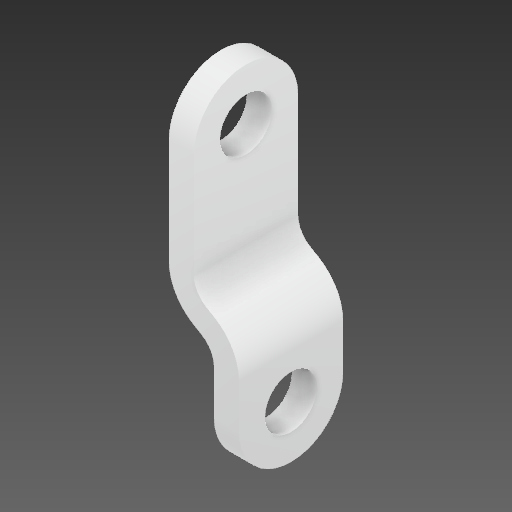
# Autodesk Inventor part: ForearmActuatorConnector2
Saved by Autodesk Inventor 2020 (Build 240168000, 168)
## iProperties
Created: 2020-04-15
Part Number: ForearmActuatorConnector2
Material: Aluminum 6061
Document SubType Name: Sheet Metal
Designer: valer
Density: 2.7 g/cm^3
Sheet Metal Rule: Default
Appearance: Aluminum - Flat
Author: valer
Autodesk Inventor part; units mm, degrees
ref_plane "YZ Plane" through (0, 0, 0) normal (1, 0, 0) x (0, 1, 0)
ref_plane "XZ Plane" through (0, 0, 0) normal (0, 1, 0) x (-1, 0, 0)
ref_plane "XY Plane" through (0, 0, 0) normal (0, 0, 1) x (1, 0, 0)
sketch "Base" plane through (0, 0, 0) normal (0, 0, 1) x (1, 0, 0)
  line L0 (0, 19.05) -> (0, -1.7843)
  line L1 (0, -1.7843) -> (5.4993, -4.9593)
  line L2 (5.4993, -4.9593) -> (5.4993, -20.1993)
  dimension "d26" = 20.8343
  dimension "d27" = 120
  dimension "d28" = 6.35
  dimension "d29" = 15.24
  measures "d26" distance of L0.start L0.end
  measures "d27" angle of L0 L1
  measures "d28" distance of L0.end L1.end
  measures "d29" distance of L1.end L2.end
contour flange "BaseFeature" sketch "Base" thickness 3.048 bend radius 3.048 width 12.7 along (0, 0, 1) mid plane no both sides no wall seen from (0, 8.6328, 0) lies toward (-1, 0, 0) curves L0 L1 L2
bend "Bend1"
corner "Corner1"
fillet "FilletsFeature" radius 6.35 4 edges at (-1.524, 19.05, 12.7) (-1.524, 19.05, 0) (3.9753, -20.1993, 12.7) (3.9753, -20.1993, 0)
sketch "ForearmHole" plane through (0, -0.0246, 12.7) normal (1, 0, 0) x (0, 0, -1)
  arc A0 (12.7, 12.7246) -> (0, 12.7246) centre (6.35, 12.7246) ccw projected
  point P0 (12.7, 0.0246)
hole "ForearmHoleFeature" at (0, 12.7, 6.35) direction (-1, 0, 0) diameter 6.35 end through all
ref_plane "MiddlePlane" through (-3.048, -0.0246, 0) normal (-1, 0, 0) x (0, 0, 1)
sketch "ActuatorMountHole" plane through (5.4993, -8.4789, 12.7) normal (1, 0, 0) x (0, 0, -1)
  arc A0 (0, -5.3705) -> (12.7, -5.3705) centre (6.35, -5.3705) ccw projected
  point P0 (12.7, 8.4789)
hole "ActuatorMountHoleFeature" at (5.4993, -13.8493, 6.35) direction (-1, 0, 0) diameter 6.35 end through all
equation "\"d17\" = Thickness"
equation "\"d36\" = Thickness"
equation "\"d0\" = Thickness"
equation "\"d1\" = BendReliefWidth"
equation "\"d2\" = BendReliefDepth"
equation "\"d3\" = MinimumRemnant"
equation "\"d4\" = TransitionRadius"
equation "\"d6\" = BendRadius"
equation "\"d8\" = CornerReliefSize"
equation "\"d9\" = GapSize"
equation "\"d10\" = JacobiRadiusSize"
equation "\"BendRadius\" = Thickness"
equation "\"BendReliefWidth\" = Thickness"
equation "\"BendReliefDepth\" = 0.5 * Thickness"
equation "\"CornerReliefSize\" = 4 * Thickness"
equation "\"MinimumRemnant\" = 2 * Thickness"
equation "\"TransitionRadius\" = BendRadius"
equation "\"JacobiRadiusSize\" = BendRadius"
equation "\"GapSize\" = Thickness"
equation "\"Thickness\" = 3.048"
body "Solid1"
